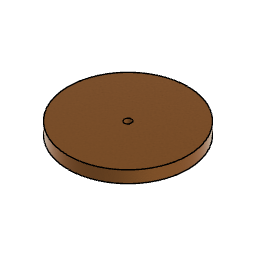
Assembly (Autodesk Fusion 360 archive; units mm, degrees)
design "ReactionWheel"
Autodesk Fusion 360 part; units mm, degrees
cylinder "CylinderPrimitive1" add diameter 100 height 10 placed x (1, 0, 0) y (0, 1, 0) z (0, 0, 1) at (0, 0, 0)
sketch "Sketch4" plane through (0, 0, 10) normal (0, 0, 1) x (-1, 0, 0)
  circle A0 centre (0, 0) radius 50
  line L0 (-2.6001, -1.4965) -> (-2.6001, 1.4965)
  arc A1 (-2.6001, -1.4965) -> (-2.6001, 1.4965) centre (0, 0) ccw
  dimension "d3" = 6
  dimension "d4" = 2.993
  constraint coincident A0.centre A1.centre
  constraint vertical L0
  measures "d3" diameter of A1
  measures "d4" distance of L0.start L0.end
extrude "Extrude1" cut sketch "Sketch4" against normal blind 10 contours L0 A1

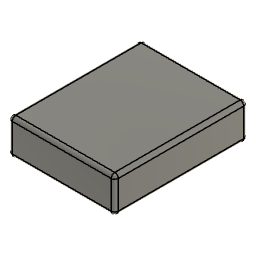
design "Battery"
Autodesk Fusion 360 part; units mm, degrees
sketch "Sketch1" plane through (0, 0, 0) normal (0, 0, 1) x (1, 0, 0)
  line L0 (-30, 37.5) -> (30, 37.5)
  line L1 (30, 37.5) -> (30, -37.5)
  line L2 (30, -37.5) -> (-30, -37.5)
  line L3 (-30, -37.5) -> (-30, 37.5)
  line L4 (-30, 37.5) -> (30, -37.5) construction
  line L5 (30, 37.5) -> (-30, -37.5) construction
  dimension "d1" = 60
  dimension "d2" = 75
  constraint horizontal L0
  constraint perpendicular L0 L1
  constraint parallel L0 L2
  constraint parallel L1 L3
  constraint coincident L4 origin
  constraint coincident L5 origin
  measures "d1" distance of L0.start L0.end
  measures "d2" distance of L0.end L1.end
extrude "Extrude1" add sketch "Sketch1" along normal blind 20
fillet "Fillet1" radius 2 12 edges at (0, -37.5, 20) (30, 0, 20) (0, 37.5, 20) (-30, 0, 20) (30, -37.5, 10) (-30, -37.5, 10) (30, 37.5, 10) (30, 0, 0) (0, -37.5, 0) (-30, 37.5, 10) (0, 37.5, 0) (-30, 0, 0)

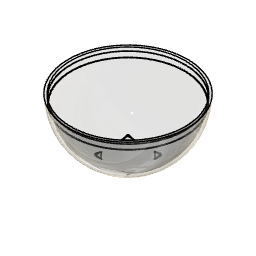
design "Sphere"
Autodesk Fusion 360 part; units mm, degrees
sketch "Sketch1" plane through (0, 0, 0) normal (1, 0, 0) x (0, 1, 0)
  arc A0 (0, 0) -> (200, 200) centre (0, 200) ccw
  line L0 (0, 0) -> (200, 0) construction
  line L1 (200, 0) -> (200, 200) construction
  line L2 (200, 200) -> (192, 200)
  line L3 (192, 200) -> (192, 188.5)
  line L4 (192, 188.5) -> (191, 188.5)
  line L5 (191, 188.5) -> (191, 171)
  line L6 (191, 171) -> (189, 171)
  arc A1 (0, 8.7881) -> (189, 171) centre (0, 200) ccw
  line L7 (0, 8.7881) -> (0, 0)
  dimension "d1" = 200
  dimension "d16" = 11.5
  dimension "d17" = 17.5
  dimension "d18" = 8
  dimension "d19" = 1
  dimension "d20" = 2
  constraint coincident A0.start L0.start
  constraint horizontal L0
  constraint tangent A0 L0
  constraint perpendicular L0 L1
  constraint tangent A0 L1
  constraint perpendicular L1 L2
  constraint perpendicular L2 L3
  constraint perpendicular L3 L4
  constraint perpendicular L4 L5
  constraint perpendicular L5 L6
  constraint coincident A0.centre A1.centre
  constraint perpendicular L0 L7
  measures "d1" distance of A0.start L0.end
  measures "d16" distance of L2.end L3.end
  measures "d17" distance of L4.end L5.end
  measures "d18" distance of A0.end L2.end
  measures "d19" distance of L3.end L4.end
  measures "d20" distance of L5.end L6.end
revolve "Revolve1" add sketch "Sketch1" angle 360 about axis through (0, 0, 1.75) along (0, 0, 1)
sketch "Sketch3" plane through (0, 0, 200) normal (0, 0, 1) x (-1, 0, 0)
  circle A0 centre (0, 0) radius 200
  line L0 (56, -56) -> (-56, -56)
  line L1 (-56, -56) -> (-56, 56)
  line L2 (-56, 56) -> (56, 56)
  line L3 (56, 56) -> (56, -56)
  line L4 (56, -56) -> (-56, 56) construction
  line L5 (-56, -56) -> (56, 56) construction
  circle A1 centre (0, 0) radius 192
  dimension "d7" = 112
  constraint horizontal L0
  constraint perpendicular L0 L1
  constraint parallel L0 L2
  constraint parallel L1 L3
  constraint coincident L4 A0.centre
  constraint coincident L5 A0.centre
  constraint coincident A0.centre A1.centre
  constraint equal L1 L2
  measures "d7" distance of L1.end L2.end
extrude "Extrude1" cut sketch "Sketch3" against normal blind 180 contours L0 L1 L2 L3
fillet "Fillet3" radius 1 4 edges at (-56, 56, 22.9799) (56, 56, 22.9799) (56, -56, 22.9799) (-56, -56, 22.9799)
